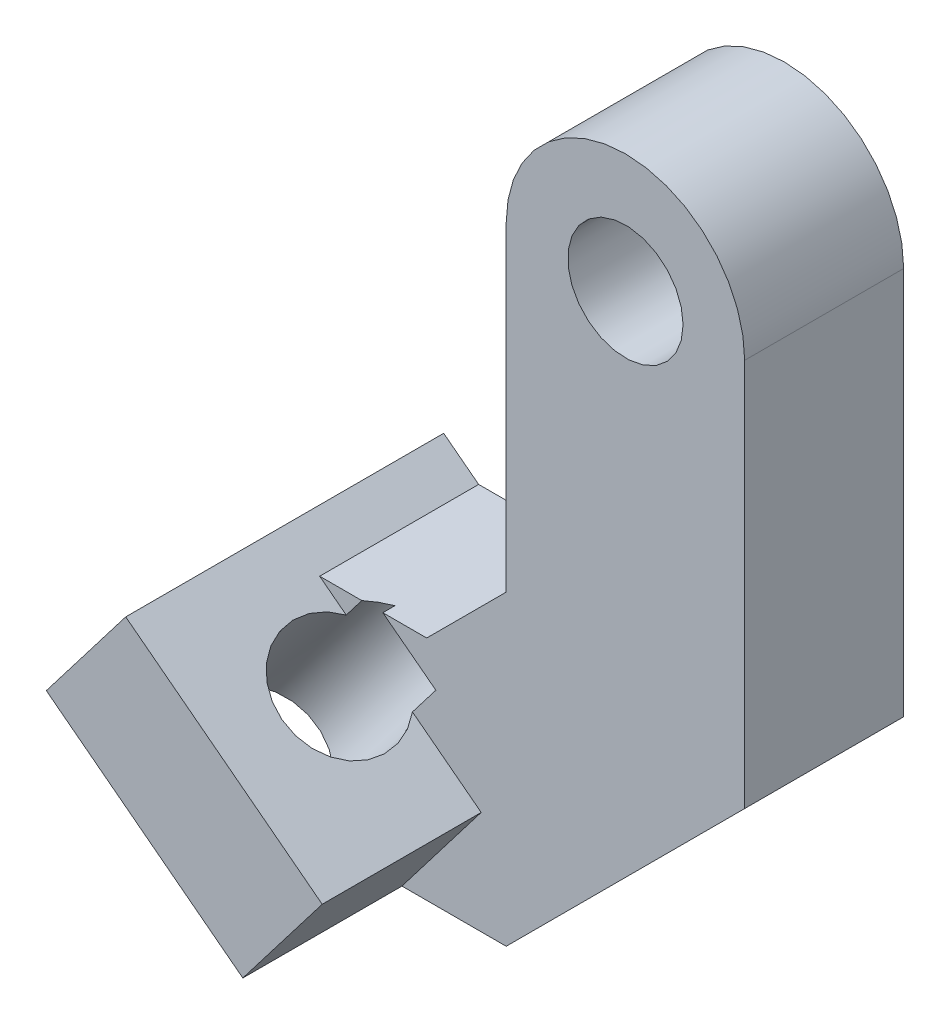
# Autodesk Inventor part: mirror_arm
Saved by Autodesk Inventor 2025.1 (Build 291241020, 241B)
## iProperties
Created: 2024-10-13
Part Number: mirror_arm
Material: Ogólny
Document SubType Name: Modeling
Designer: zychlix
Density: 1 g/cm^3
Appearance: Domyślna
Author: zychlix
Autodesk Inventor part; units mm, degrees
ref_plane "YZ Plane" through (0, 0, 0) normal (1, 0, 0) x (0, 1, 0)
ref_plane "XZ Plane" through (0, 0, 0) normal (0, 1, 0) x (-1, 0, 0)
ref_plane "XY Plane" through (0, 0, 0) normal (0, 0, 1) x (1, 0, 0)
sketch "Szkic1" plane through (0, 0, 0) normal (0, 0, 1) x (1, 0, 0)
  circle A0 centre (26.2, 0.975) radius 1.45 projected
  circle A1 centre (26.2, 0.975) radius 3
  line L0 (29.2, 0.975) -> (29.2, -8.7925)
  line L1 (23.2, -14.7925) -> (20.5681, -14.7925)
  line L2 (17.1107, -9.0757) -> (21.2, -9.0757)
  line L3 (23.2, -7.0757) -> (23.2, 0.975)
  line L4 (18.2447, -12.1144) -> (21.525, -14.6291)
  line L5 (16.8275, -11.925) -> (-16.8275, 13.875) construction
  line L6 (20.0699, -9.7335) -> (23.3502, -12.2482)
  line L7 (18.2447, -12.1144) -> (20.0699, -9.7335)
  line L8 (21.525, -14.6291) -> (23.3502, -12.2482)
  line L9 (29.2, -8.7925) -> (23.2, -14.7925)
  line L10 (15.6301, -11.0071) -> (17.1107, -9.0757)
  line L11 (21.2, -9.0757) -> (23.2, -7.0757)
  line L12 (15.6301, -11.0071) -> (20.5681, -14.7925)
  point P0 (0, 0)
  point P1 (29.2, -14.7925)
  point P2 (18.5681, -14.7925)
  point P3 (15.1107, -9.0757)
  point P4 (23.2, -9.0757)
  point P5 (18.9313, -9.4578)
  point P6 (19.7101, -9.4578)
  dimension "d0" = 3
  dimension "d5" = 6
  dimension "d6" = 6
  dimension "d7" = 2
  dimension "d9" = 2
  dimension "d10" = 2
  dimension "d11" = 2
  dimension "d12" = 2
  dimension "d13" = 6
  constraints: 25 end point, 6 point on line, 3 parallel, 3 perpendicular, 2 collinear, 2 point on circle, 2 tangent, 1 centre point, 1 coincident, 1 vertical
  measures "d0" distance of L4.end L6.end
  measures "d5" distance of L0.end point (29.2, -14.793)
  measures "d6" distance of L1.start point (29.2, -14.793)
  measures "d7" distance of L1.end point (18.568, -14.793)
  measures "d9" distance of L10.start point (15.111, -9.076)
  measures "d10" distance of L2.start point (15.111, -9.076)
  measures "d11" distance of L2.end point (23.2, -9.076)
  measures "d12" distance of L3.start point (23.2, -9.076)
  measures "d13" diameter of A1
extrude "Wyciągnięcie proste1" add sketch "Szkic1" along normal blind 4 contours A1 | L0 L9 L1 L12 L10 L2 L11 L3 A1 | L7 L6 L8 L4
sketch "Szkic4" plane through (0, 0, 4) normal (0, 0, 1) x (1, 0, 0)
  line L0 (22.5711, -12.1912) -> (17.6276, -8.4015)
  line L1 (16.8275, -11.925) -> (-16.8275, 13.875) construction
  line L2 (17.6276, -8.4015) -> (15.6301, -11.0071)
  line L3 (15.6301, -11.0071) -> (20.5737, -14.7968)
  line L4 (20.5737, -14.7968) -> (22.5711, -12.1912)
  line L5 (15.6301, -11.0071) -> (20.5681, -14.7925) projected
  line L6 (17.1107, -9.0757) -> (15.6301, -11.0071) projected
  point P0 (0, 0)
  constraints: 8 end point, 2 collinear, 2 perpendicular, 1 parallel
extrude "Wyciągnięcie proste2" add sketch "Szkic4" along normal blind 4 and the other way blind 4
sketch "Szkic5" plane through (20.5737, -14.7968, 0) normal (-0.6084, -0.7936, 0) x (0.7936, -0.6084, 0)
  circle A0 centre (-3.229, 5) radius 1.45
  line L0 (-6.229, 0) -> (-6.229, 8) projected
  line L1 (-6.229, 8) -> (0, 8) projected
  point P0 (-25.3303, 0)
  dimension "d16" = 3
  dimension "d17" = 3
  dimension "d18" = 2.9
  constraints: 1 centre point
  measures "d16" distance from line of L0 A0.centre
  measures "d17" distance from line of L1 A0.centre
  measures "d18" diameter of A0
extrude "Wyciągnięcie proste3" cut sketch "Szkic5" against normal blind 4.25
equation "\"d6\" = d5"
equation "\"d9\" = d7"
equation "\"d10\" = d9"
equation "\"d11\" = d7"
equation "\"d12\" = d11"
